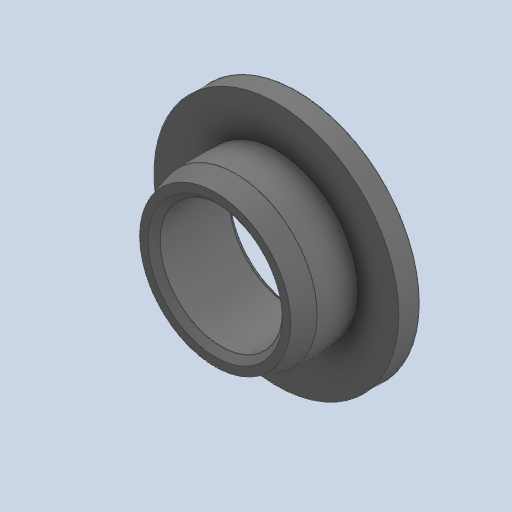
# Autodesk Inventor part: 80F-0603
Saved by Autodesk Inventor 2022 (Build 260153000, 153)
## iProperties
Part Number: 80F-0603
Material: 一般
Document SubType Name: Modeling
Designer: Masato Kubotera
Density: 1.2841 g/cm^3
Appearance: 灰色
Catalog Web Link: https://jp.misumi-ec.com/vona2/detail/221000090789/?HissuCode=80F-0603
Mass: 0.186667 g
Surface Area: 3.44616 cm^2
Volume: 0.145368 cm^3
Description: ReadyMade
Author: Masato Kubotera
Autodesk Inventor part; units mm, degrees
ref_plane "YZ Plane" through (0, 0, 0) normal (1, 0, 0) x (0, 1, 0)
ref_plane "XZ Plane" through (0, 0, 0) normal (0, 1, 0) x (-1, 0, 0)
ref_plane "XY Plane" through (0, 0, 0) normal (0, 0, 1) x (1, 0, 0)
sketch "スケッチ1" plane through (0, 0, 0) normal (0, 1, 0) x (-1, 0, 0)
  line L0 (-3, 0.3) -> (-3, 3.7)
  line L1 (-3.3, 4) -> (-3.7, 4)
  line L2 (-4, 3) -> (-4, 1)
  line L3 (-4, 1) -> (-6, 1)
  line L4 (-6, 1) -> (-6, 0)
  line L5 (-6, 0) -> (-3.3, 0)
  line L6 (-3, 3.7) -> (-3.3, 4)
  line L7 (-3, 0.3) -> (-3.3, 0)
  line L8 (-3.7, 4) -> (-4, 3)
  line L9 (0, -0.8) -> (0, 4.8) projected
  point P0 (0, 0)
  point P1 (-3, 0)
  point P2 (-3, 4)
  point P3 (-4, 4)
  dimension "d2" = 1
  dimension "d9" = 1
  dimension "d11" = 6
  dimension "d12" = 8
  dimension "d13" = 12
  dimension "d14" = 0.3
  dimension "d15" = 0.3
  dimension "d16" = 0.3
  dimension "d17" = 0.3
  dimension "d18" = 0.3
  dimension "d19" = 4
  constraints: 18 end point, 7 point on line, 4 perpendicular, 2 parallel, 1 vertical
  measures "d2" distance of L3.end L4.end
  measures "d9" distance of L2.start point (-4, 4)
  measures "d11" diameter of L0 L9
  measures "d12" diameter of L2 L9
  measures "d13" diameter of L4 L9
  measures "d14" distance from line of L0.start L5
  measures "d15" distance from line of L5.end L0
  measures "d16" distance from line of L0.end L1
  measures "d17" horizontal distance of L0.end L1.start
  measures "d18" distance from line of L2 L1.end
  measures "d19" distance of point (-3, 4) point (-3, 0)
revolve "回転1" add sketch "スケッチ1" angle 360 about axis through (0, 0, -10) along (0, 0, 1)
equation "\"d15\" = d14"
equation "\"d16\" = d14"
equation "\"d17\" = d16"
equation "\"d18\" = d14"
